Autodesk Inventor part; units mm, degrees
(part 3 of 3)
sketch "Sketch16" plane through (-107.75, 0, 0) normal (0, 0, 1) x (1, 0, 0)
  line L0 (4.2221, 29.7336) -> (86.2779, 29.7336) construction
  line L1 (86.2779, 29.7336) -> (86.2779, 24.45) construction
  line L2 (86.2779, 24.45) -> (4.2221, 24.45) construction
  line L3 (4.2221, 24.45) -> (4.2221, 29.7336) construction
  line L4 (30.85, 22.45) -> (59.65, 22.45) projected
  line L5 (20.4356, 29.4257) -> (17.6446, 29.4257)
  line L6 (17.6446, 29.4257) -> (17.6446, 27.7336)
  line L7 (17.6446, 27.7336) -> (20.3189, 27.7336)
  line L8 (20.3189, 27.7336) -> (20.3189, 27.0237)
  line L9 (20.3189, 27.0237) -> (17.6446, 27.0237)
  line L10 (17.6446, 27.0237) -> (17.6446, 24.1356)
  line L11 (17.6446, 24.1356) -> (16.8472, 24.1356)
  line L12 (16.8472, 24.1356) -> (16.8472, 30.1356)
  line L13 (16.8472, 30.1356) -> (20.4356, 30.1356)
  line L14 (20.4356, 30.1356) -> (20.4356, 29.4257)
  line L15 (23.4793, 27.826) -> (23.4404, 27.826)
  spline S0 degree 2 poles (23.4404, 27.826) (23.3529, 27.8503) (23.1633, 27.86) (23.032, 27.86) knots 0 0 0 1 2 2 2
  spline S1 degree 2 poles (23.032, 27.86) (22.7257, 27.86) (22.1228, 27.5926) (21.8505, 27.3301) knots 0 0 0 1 2 2 2
  line L16 (21.8505, 27.3301) -> (21.8505, 24.1356)
  line L17 (21.8505, 24.1356) -> (21.092, 24.1356)
  line L18 (21.092, 24.1356) -> (21.092, 28.638)
  line L19 (21.092, 28.638) -> (21.8505, 28.638)
  line L20 (21.8505, 28.638) -> (21.8505, 27.967)
  spline S2 degree 2 poles (21.8505, 27.967) (22.2638, 28.3365) (22.8813, 28.638) (23.173, 28.638) knots 0 0 0 1 2 2 2
  spline S3 degree 2 poles (23.173, 28.638) (23.2897, 28.638) (23.4064, 28.6283) (23.4793, 28.6137) knots 0 0 0 1 2 2 2
  line L21 (23.4793, 28.6137) -> (23.4793, 27.826)
  spline S4 degree 2 poles (27.7678, 26.3868) (27.7678, 25.249) (26.6738, 24.0092) (25.7597, 24.0092) knots 0 0 0 1 2 2 2
  spline S5 degree 2 poles (25.7597, 24.0092) (24.8213, 24.0092) (23.7468, 25.2879) (23.7468, 26.3868) knots 0 0 0 1 2 2 2
  spline S6 degree 2 poles (23.7468, 26.3868) (23.7468, 27.5148) (24.8553, 28.7644) (25.7597, 28.7644) knots 0 0 0 1 2 2 2
  spline S7 degree 2 poles (25.7597, 28.7644) (26.6738, 28.7644) (27.7678, 27.5197) (27.7678, 26.3868) knots 0 0 0 1 2 2 2
  spline S8 degree 2 poles (26.985, 26.3868) (26.985, 27.262) (26.3481, 28.1129) (25.7597, 28.1129) knots 0 0 0 1 2 2 2
  spline S9 degree 2 poles (25.7597, 28.1129) (25.1714, 28.1129) (24.5296, 27.262) (24.5296, 26.3868) knots 0 0 0 1 2 2 2
  spline S10 degree 2 poles (24.5296, 26.3868) (24.5296, 25.5359) (25.1714, 24.6607) (25.7597, 24.6607) knots 0 0 0 1 2 2 2
  spline S11 degree 2 poles (25.7597, 24.6607) (26.3432, 24.6607) (26.985, 25.5213) (26.985, 26.3868) knots 0 0 0 1 2 2 2
  line L22 (32.0806, 24.1356) -> (31.3221, 24.1356)
  line L23 (31.3221, 24.1356) -> (31.3221, 26.7028)
  spline S12 degree 2 poles (31.3221, 26.7028) (31.3221, 27.014) (31.2638, 27.5489) (31.1763, 27.7093) knots 0 0 0 1 2 2 2
  spline S13 degree 2 poles (31.1763, 27.7093) (31.0839, 27.8795) (30.7532, 28.0448) (30.4712, 28.0448) knots 0 0 0 1 2 2 2
  spline S14 degree 2 poles (30.4712, 28.0448) (30.1892, 28.0448) (29.5912, 27.7434) (29.3043, 27.5002) knots 0 0 0 1 2 2 2
  line L24 (29.3043, 27.5002) -> (29.3043, 24.1356)
  line L25 (29.3043, 24.1356) -> (28.5458, 24.1356)
  line L26 (28.5458, 24.1356) -> (28.5458, 28.638)
  line L27 (28.5458, 28.638) -> (29.3043, 28.638)
  line L28 (29.3043, 28.638) -> (29.3043, 28.1372)
  spline S15 degree 2 poles (29.3043, 28.1372) (29.6447, 28.4435) (30.3011, 28.7644) (30.6706, 28.7644) knots 0 0 0 1 2 2 2
  spline S16 degree 2 poles (30.6706, 28.7644) (31.3318, 28.7644) (32.0806, 27.8892) (32.0806, 27.0578) knots 0 0 0 1 2 2 2
  line L29 (32.0806, 27.0578) -> (32.0806, 24.1356)
  spline S17 degree 2 poles (34.5069, 24.0481) (33.8894, 24.0481) (33.1941, 24.7531) (33.1941, 25.5165) knots 0 0 0 1 2 2 2
  line L30 (33.1941, 25.5165) -> (33.1941, 28.0108)
  line L31 (33.1941, 28.0108) -> (32.6835, 28.0108)
  line L32 (32.6835, 28.0108) -> (32.6835, 28.638)
  line L33 (32.6835, 28.638) -> (33.1941, 28.638)
  line L34 (33.1941, 28.638) -> (33.1941, 29.9314)
  line L35 (33.1941, 29.9314) -> (33.9526, 29.9314)
  line L36 (33.9526, 29.9314) -> (33.9526, 28.638)
  line L37 (33.9526, 28.638) -> (35.3481, 28.638)
  line L38 (35.3481, 28.638) -> (35.3481, 28.0108)
  line L39 (35.3481, 28.0108) -> (33.9526, 28.0108)
  line L40 (33.9526, 28.0108) -> (33.9526, 25.8665)
  spline S18 degree 2 poles (33.9526, 25.8665) (33.9526, 25.5262) (33.9769, 25.1518) (34.0596, 24.9913) knots 0 0 0 1 2 2 2
  spline S19 degree 2 poles (34.0596, 24.9913) (34.1276, 24.8503) (34.434, 24.7093) (34.6965, 24.7093) knots 0 0 0 1 2 2 2
  spline S20 degree 2 poles (34.6965, 24.7093) (34.8813, 24.7093) (35.2265, 24.8212) (35.3043, 24.8552) knots 0 0 0 1 2 2 2
  line L41 (35.3043, 24.8552) -> (35.3481, 24.8552)
  line L42 (35.3481, 24.8552) -> (35.3481, 24.1745)
  spline S21 degree 2 poles (35.3481, 24.1745) (35.1341, 24.1161) (34.6965, 24.0481) (34.5069, 24.0481) knots 0 0 0 1 2 2 2
  spline S22 degree 2 poles (42.6122, 25.9784) (42.6122, 25.531) (42.2719, 24.8455) (41.9899, 24.6218) knots 0 0 0 1 2 2 2
  spline S23 degree 2 poles (41.9899, 24.6218) (41.6495, 24.3592) (40.8764, 24.1356) (40.2638, 24.1356) knots 0 0 0 1 2 2 2
  line L43 (40.2638, 24.1356) -> (38.5425, 24.1356)
  line L44 (38.5425, 24.1356) -> (38.5425, 30.1356)
  line L45 (38.5425, 30.1356) -> (40.1325, 30.1356)
  spline S24 degree 2 poles (40.1325, 30.1356) (40.7743, 30.1356) (41.4161, 30.0529) (41.7079, 29.8925) knots 0 0 0 1 2 2 2
  spline S25 degree 2 poles (41.7079, 29.8925) (42.0336, 29.7223) (42.3302, 29.1631) (42.3302, 28.7839) knots 0 0 0 1 2 2 2
  spline S26 degree 2 poles (42.3302, 28.7839) (42.3302, 28.3609) (41.8829, 27.6899) (41.4891, 27.5002) knots 0 0 0 1 2 2 2
  line L46 (41.4891, 27.5002) -> (41.4891, 27.4711)
  spline S27 degree 2 poles (41.4891, 27.4711) (42.0239, 27.3252) (42.6122, 26.5521) (42.6122, 25.9784) knots 0 0 0 1 2 2 2
  spline S28 degree 2 poles (41.7808, 25.9443) (41.7808, 26.2847) (41.5863, 26.7223) (41.2946, 26.8779) knots 0 0 0 1 2 2 2
  spline S29 degree 2 poles (41.2946, 26.8779) (41.1049, 26.9751) (40.6576, 27.0335) (40.2443, 27.0335) knots 0 0 0 1 2 2 2
  line L47 (40.2443, 27.0335) -> (39.34, 27.0335)
  line L48 (39.34, 27.0335) -> (39.34, 24.8163)
  line L49 (39.34, 24.8163) -> (39.9866, 24.8163)
  spline S30 degree 2 poles (39.9866, 24.8163) (40.5117, 24.8163) (41.1147, 24.9135) (41.3481, 25.0691) knots 0 0 0 1 2 2 2
  spline S31 degree 2 poles (41.3481, 25.0691) (41.5717, 25.2296) (41.7808, 25.6283) (41.7808, 25.9443) knots 0 0 0 1 2 2 2
  spline S32 degree 2 poles (41.4988, 28.672) (41.4988, 28.886) (41.3529, 29.2069) (41.1925, 29.2993) knots 0 0 0 1 2 2 2
  spline S33 degree 2 poles (41.1925, 29.2993) (40.998, 29.4062) (40.5263, 29.4549) (40.1033, 29.4549) knots 0 0 0 1 2 2 2
  line L50 (40.1033, 29.4549) -> (39.34, 29.4549)
  line L51 (39.34, 29.4549) -> (39.34, 27.6996)
  line L52 (39.34, 27.6996) -> (40.2443, 27.6996)
  spline S34 degree 2 poles (40.2443, 27.6996) (40.6187, 27.6996) (40.9737, 27.7774) (41.1633, 27.8989) knots 0 0 0 1 2 2 2
  spline S35 degree 2 poles (41.1633, 27.8989) (41.3481, 28.0156) (41.4988, 28.39) (41.4988, 28.672) knots 0 0 0 1 2 2 2
  spline S36 degree 2 poles (47.0466, 26.3868) (47.0466, 25.249) (45.9526, 24.0092) (45.0385, 24.0092) knots 0 0 0 1 2 2 2
  spline S37 degree 2 poles (45.0385, 24.0092) (44.1001, 24.0092) (43.0255, 25.2879) (43.0255, 26.3868) knots 0 0 0 1 2 2 2
  spline S38 degree 2 poles (43.0255, 26.3868) (43.0255, 27.5148) (44.1341, 28.7644) (45.0385, 28.7644) knots 0 0 0 1 2 2 2
  spline S39 degree 2 poles (45.0385, 28.7644) (45.9526, 28.7644) (47.0466, 27.5197) (47.0466, 26.3868) knots 0 0 0 1 2 2 2
  spline S40 degree 2 poles (46.2638, 26.3868) (46.2638, 27.262) (45.6268, 28.1129) (45.0385, 28.1129) knots 0 0 0 1 2 2 2
  spline S41 degree 2 poles (45.0385, 28.1129) (44.4502, 28.1129) (43.8083, 27.262) (43.8083, 26.3868) knots 0 0 0 1 2 2 2
  spline S42 degree 2 poles (43.8083, 26.3868) (43.8083, 25.5359) (44.4502, 24.6607) (45.0385, 24.6607) knots 0 0 0 1 2 2 2
  spline S43 degree 2 poles (45.0385, 24.6607) (45.622, 24.6607) (46.2638, 25.5213) (46.2638, 26.3868) knots 0 0 0 1 2 2 2
  line L53 (51.3205, 24.1356) -> (50.3918, 24.1356)
  line L54 (50.3918, 24.1356) -> (49.2978, 25.8276)
  line L55 (49.2978, 25.8276) -> (48.1746, 24.1356)
  line L56 (48.1746, 24.1356) -> (47.314, 24.1356)
  line L57 (47.314, 24.1356) -> (48.8748, 26.3673)
  line L58 (48.8748, 26.3673) -> (47.3286, 28.638)
  line L59 (47.3286, 28.638) -> (48.2573, 28.638)
  line L60 (48.2573, 28.638) -> (49.3464, 26.9605)
  line L61 (49.3464, 26.9605) -> (50.4599, 28.638)
  line L62 (50.4599, 28.638) -> (51.3205, 28.638)
  line L63 (51.3205, 28.638) -> (49.7694, 26.416)
  line L64 (49.7694, 26.416) -> (51.3205, 24.1356)
  line L65 (61.2686, 30.1356) -> (59.7613, 24.1356)
  line L66 (59.7613, 24.1356) -> (58.8667, 24.1356)
  line L67 (58.8667, 24.1356) -> (57.6463, 29.1145)
  line L68 (57.6463, 29.1145) -> (56.4599, 24.1356)
  line L69 (56.4599, 24.1356) -> (55.575, 24.1356)
  line L70 (55.575, 24.1356) -> (54.0434, 30.1356)
  line L71 (54.0434, 30.1356) -> (54.8651, 30.1356)
  line L72 (54.8651, 30.1356) -> (56.0709, 25.1615)
  line L73 (56.0709, 25.1615) -> (57.267, 30.1356)
  line L74 (57.267, 30.1356) -> (58.079, 30.1356)
  line L75 (58.079, 30.1356) -> (59.2848, 25.1032)
  line L76 (59.2848, 25.1032) -> (60.4858, 30.1356)
  line L77 (60.4858, 30.1356) -> (61.2686, 30.1356)
  line L78 (62.6981, 24.1356) -> (61.9396, 24.1356)
  line L79 (61.9396, 24.1356) -> (61.9396, 28.638)
  line L80 (61.9396, 28.638) -> (62.6981, 28.638)
  line L81 (62.6981, 28.638) -> (62.6981, 24.1356)
  line L82 (62.7516, 29.3868) -> (61.891, 29.3868)
  line L83 (61.891, 29.3868) -> (61.891, 30.1745)
  line L84 (61.891, 30.1745) -> (62.7516, 30.1745)
  line L85 (62.7516, 30.1745) -> (62.7516, 29.3868)
  line L86 (66.1989, 27.826) -> (66.16, 27.826)
  spline S44 degree 2 poles (66.16, 27.826) (66.0725, 27.8503) (65.8829, 27.86) (65.7516, 27.86) knots 0 0 0 1 2 2 2
  spline S45 degree 2 poles (65.7516, 27.86) (65.4453, 27.86) (64.8424, 27.5926) (64.5701, 27.3301) knots 0 0 0 1 2 2 2
  line L87 (64.5701, 27.3301) -> (64.5701, 24.1356)
  line L88 (64.5701, 24.1356) -> (63.8116, 24.1356)
  line L89 (63.8116, 24.1356) -> (63.8116, 28.638)
  line L90 (63.8116, 28.638) -> (64.5701, 28.638)
  line L91 (64.5701, 28.638) -> (64.5701, 27.967)
  spline S46 degree 2 poles (64.5701, 27.967) (64.9834, 28.3365) (65.6009, 28.638) (65.8926, 28.638) knots 0 0 0 1 2 2 2
  spline S47 degree 2 poles (65.8926, 28.638) (66.0093, 28.638) (66.126, 28.6283) (66.1989, 28.6137) knots 0 0 0 1 2 2 2
  line L92 (66.1989, 28.6137) -> (66.1989, 27.826)
  spline S48 degree 2 poles (68.7419, 24.0335) (67.6625, 24.0335) (66.4761, 25.2442) (66.4761, 26.3625) knots 0 0 0 1 2 2 2
  spline S49 degree 2 poles (66.4761, 26.3625) (66.4761, 27.4613) (67.6284, 28.7644) (68.5571, 28.7644) knots 0 0 0 1 2 2 2
  spline S50 degree 2 poles (68.5571, 28.7644) (68.9753, 28.7644) (69.622, 28.5213) (69.8602, 28.2636) knots 0 0 0 1 2 2 2
  spline S51 degree 2 poles (69.8602, 28.2636) (70.1033, 28.0059) (70.361, 27.262) (70.361, 26.7223) knots 0 0 0 1 2 2 2
  line L93 (70.361, 26.7223) -> (70.361, 26.309)
  line L94 (70.361, 26.309) -> (67.2443, 26.309)
  spline S52 degree 2 poles (67.2443, 26.309) (67.2443, 25.5262) (68.032, 24.6947) (68.7322, 24.6947) knots 0 0 0 1 2 2 2
  spline S53 degree 2 poles (68.7322, 24.6947) (68.9801, 24.6947) (69.4615, 24.8066) (69.656, 24.8941) knots 0 0 0 1 2 2 2
  spline S54 degree 2 poles (69.656, 24.8941) (69.8602, 24.9913) (70.1422, 25.1615) (70.2346, 25.2393) knots 0 0 0 1 2 2 2
  line L95 (70.2346, 25.2393) -> (70.2784, 25.2393)
  line L96 (70.2784, 25.2393) -> (70.2784, 24.4127)
  spline S55 degree 2 poles (70.2784, 24.4127) (70.1471, 24.3592) (69.7484, 24.2036) (69.5928, 24.1599) knots 0 0 0 1 2 2 2
  spline S56 degree 2 poles (69.5928, 24.1599) (69.374, 24.0967) (69.0142, 24.0335) (68.7419, 24.0335) knots 0 0 0 1 2 2 2
  spline S57 degree 2 poles (69.622, 26.8876) (69.6122, 27.1939) (69.4858, 27.6412) (69.3643, 27.792) knots 0 0 0 1 2 2 2
  spline S58 degree 2 poles (69.3643, 27.792) (69.233, 27.9622) (68.8197, 28.1421) (68.5134, 28.1421) knots 0 0 0 1 2 2 2
  spline S59 degree 2 poles (68.5134, 28.1421) (68.2119, 28.1421) (67.7889, 27.9622) (67.6139, 27.7871) knots 0 0 0 1 2 2 2
  spline S60 degree 2 poles (67.6139, 27.7871) (67.4437, 27.6072) (67.2686, 27.1745) (67.2443, 26.8876) knots 0 0 0 1 2 2 2
  line L97 (67.2443, 26.8876) -> (69.622, 26.8876)
  spline S61 degree 2 poles (72.3448, 24.0286) (71.8926, 24.0286) (71.1098, 24.2717) (70.8521, 24.4079) knots 0 0 0 1 2 2 2
  line L98 (70.8521, 24.4079) -> (70.8521, 25.2588)
  line L99 (70.8521, 25.2588) -> (70.891, 25.2588)
  spline S62 degree 2 poles (70.891, 25.2588) (70.9882, 25.181) (71.2508, 24.9962) (71.4696, 24.8941) knots 0 0 0 1 2 2 2
  spline S63 degree 2 poles (71.4696, 24.8941) (71.6592, 24.8017) (72.126, 24.6656) (72.374, 24.6656) knots 0 0 0 1 2 2 2
  spline S64 degree 2 poles (72.374, 24.6656) (72.5539, 24.6656) (72.9672, 24.7482) (73.0644, 24.8163) knots 0 0 0 1 2 2 2
  spline S65 degree 2 poles (73.0644, 24.8163) (73.2054, 24.9087) (73.3318, 25.1177) (73.3318, 25.3317) knots 0 0 0 1 2 2 2
  spline S66 degree 2 poles (73.3318, 25.3317) (73.3318, 25.5991) (73.0401, 25.8763) (72.6657, 25.9686) knots 0 0 0 1 2 2 2
  spline S67 degree 2 poles (72.6657, 25.9686) (72.5199, 26.0027) (72.0531, 26.0999) (71.8537, 26.1534) knots 0 0 0 1 2 2 2
  spline S68 degree 2 poles (71.8537, 26.1534) (71.3383, 26.3041) (70.8716, 26.9265) (70.8716, 27.369) knots 0 0 0 1 2 2 2
  spline S69 degree 2 poles (70.8716, 27.369) (70.8716, 27.9816) (71.7905, 28.745) (72.549, 28.745) knots 0 0 0 1 2 2 2
  spline S70 degree 2 poles (72.549, 28.745) (72.9234, 28.745) (73.6819, 28.5602) (73.9396, 28.4192) knots 0 0 0 1 2 2 2
  line L100 (73.9396, 28.4192) -> (73.9396, 27.6072)
  line L101 (73.9396, 27.6072) -> (73.9007, 27.6072)
  spline S71 degree 2 poles (73.9007, 27.6072) (73.609, 27.8406) (72.8991, 28.108) (72.5344, 28.108) knots 0 0 0 1 2 2 2
  spline S72 degree 2 poles (72.5344, 28.108) (72.16, 28.108) (71.6447, 27.792) (71.6447, 27.4759) knots 0 0 0 1 2 2 2
  spline S73 degree 2 poles (71.6447, 27.4759) (71.6447, 27.1891) (71.951, 26.9119) (72.2913, 26.8244) knots 0 0 0 1 2 2 2
  spline S74 degree 2 poles (72.2913, 26.8244) (72.4566, 26.7806) (72.8748, 26.6931) (73.1033, 26.6396) knots 0 0 0 1 2 2 2
  spline S75 degree 2 poles (73.1033, 26.6396) (73.5993, 26.5132) (74.1049, 25.9346) (74.1049, 25.4338) knots 0 0 0 1 2 2 2
  spline S76 degree 2 poles (74.1049, 25.4338) (74.1049, 25.1421) (73.8764, 24.6267) (73.6528, 24.437) knots 0 0 0 1 2 2 2
  spline S77 degree 2 poles (73.6528, 24.437) (73.4145, 24.2377) (72.8067, 24.0286) (72.3448, 24.0286) knots 0 0 0 1 2 2 2
  point P0 (107.75, 0)
  point P1 (45.25, 24.45)
  point P2 (45.25, 22.45)
  point P3 (45.25, 22.45)
  dimension "d146" = 0
  dimension "d147" = 2
  constraints: 3 midpoint, 2 other
  measures "d146" horizontal distance of point (45.25, 24.45) point (45.25, 22.45)
  measures "d147" distance of point (45.25, 22.45) point (45.25, 24.45)
sketch "Sketch17" plane through (0, 0, -2.25) normal (1, 0, 0) x (0, 0, -1)
  line L0 (72.0372, 28.5438) -> (116.4628, 28.5438) construction
  line L1 (116.4628, 28.5438) -> (116.4628, 24.45) construction
  line L2 (116.4628, 24.45) -> (72.0372, 24.45) construction
  line L3 (72.0372, 24.45) -> (72.0372, 28.5438) construction
  line L4 (88.9, 22.45) -> (99.6, 22.45) projected
  line L5 (78.0247, 23.5407) -> (77.2273, 23.5407)
  line L6 (77.2273, 23.5407) -> (77.2273, 28.7092)
  line L7 (77.2273, 28.7092) -> (75.6617, 25.1938)
  line L8 (75.6617, 25.1938) -> (75.1754, 25.1938)
  line L9 (75.1754, 25.1938) -> (73.6244, 28.7092)
  line L10 (73.6244, 28.7092) -> (73.6244, 23.5407)
  line L11 (73.6244, 23.5407) -> (72.8805, 23.5407)
  line L12 (72.8805, 23.5407) -> (72.8805, 29.5407)
  line L13 (72.8805, 29.5407) -> (73.9696, 29.5407)
  line L14 (73.9696, 29.5407) -> (75.4672, 26.2003)
  line L15 (75.4672, 26.2003) -> (76.9161, 29.5407)
  line L16 (76.9161, 29.5407) -> (78.0247, 29.5407)
  line L17 (78.0247, 29.5407) -> (78.0247, 23.5407)
  spline S0 degree 2 poles (82.8821, 25.7919) (82.8821, 24.6541) (81.7881, 23.4143) (80.874, 23.4143) knots 0 0 0 1 2 2 2
  spline S1 degree 2 poles (80.874, 23.4143) (79.9356, 23.4143) (78.861, 24.693) (78.861, 25.7919) knots 0 0 0 1 2 2 2
  spline S2 degree 2 poles (78.861, 25.7919) (78.861, 26.9199) (79.9696, 28.1695) (80.874, 28.1695) knots 0 0 0 1 2 2 2
  spline S3 degree 2 poles (80.874, 28.1695) (81.7881, 28.1695) (82.8821, 26.9248) (82.8821, 25.7919) knots 0 0 0 1 2 2 2
  spline S4 degree 2 poles (82.0993, 25.7919) (82.0993, 26.6671) (81.4623, 27.518) (80.874, 27.518) knots 0 0 0 1 2 2 2
  spline S5 degree 2 poles (80.874, 27.518) (80.2857, 27.518) (79.6438, 26.6671) (79.6438, 25.7919) knots 0 0 0 1 2 2 2
  spline S6 degree 2 poles (79.6438, 25.7919) (79.6438, 24.941) (80.2857, 24.0658) (80.874, 24.0658) knots 0 0 0 1 2 2 2
  spline S7 degree 2 poles (80.874, 24.0658) (81.4575, 24.0658) (82.0993, 24.9264) (82.0993, 25.7919) knots 0 0 0 1 2 2 2
  spline S8 degree 2 poles (85.0215, 23.4532) (84.404, 23.4532) (83.7087, 24.1582) (83.7087, 24.9216) knots 0 0 0 1 2 2 2
  line L18 (83.7087, 24.9216) -> (83.7087, 27.4159)
  line L19 (83.7087, 27.4159) -> (83.1981, 27.4159)
  line L20 (83.1981, 27.4159) -> (83.1981, 28.0431)
  line L21 (83.1981, 28.0431) -> (83.7087, 28.0431)
  line L22 (83.7087, 28.0431) -> (83.7087, 29.3365)
  line L23 (83.7087, 29.3365) -> (84.4672, 29.3365)
  line L24 (84.4672, 29.3365) -> (84.4672, 28.0431)
  line L25 (84.4672, 28.0431) -> (85.8626, 28.0431)
  line L26 (85.8626, 28.0431) -> (85.8626, 27.4159)
  line L27 (85.8626, 27.4159) -> (84.4672, 27.4159)
  line L28 (84.4672, 27.4159) -> (84.4672, 25.2716)
  spline S9 degree 2 poles (84.4672, 25.2716) (84.4672, 24.9313) (84.4915, 24.5569) (84.5741, 24.3964) knots 0 0 0 1 2 2 2
  spline S10 degree 2 poles (84.5741, 24.3964) (84.6422, 24.2554) (84.9485, 24.1144) (85.2111, 24.1144) knots 0 0 0 1 2 2 2
  spline S11 degree 2 poles (85.2111, 24.1144) (85.3959, 24.1144) (85.7411, 24.2263) (85.8189, 24.2603) knots 0 0 0 1 2 2 2
  line L29 (85.8189, 24.2603) -> (85.8626, 24.2603)
  line L30 (85.8626, 24.2603) -> (85.8626, 23.5796)
  spline S12 degree 2 poles (85.8626, 23.5796) (85.6487, 23.5212) (85.2111, 23.4532) (85.0215, 23.4532) knots 0 0 0 1 2 2 2
  spline S13 degree 2 poles (90.122, 25.7919) (90.122, 24.6541) (89.028, 23.4143) (88.1139, 23.4143) knots 0 0 0 1 2 2 2
  spline S14 degree 2 poles (88.1139, 23.4143) (87.1754, 23.4143) (86.1009, 24.693) (86.1009, 25.7919) knots 0 0 0 1 2 2 2
  spline S15 degree 2 poles (86.1009, 25.7919) (86.1009, 26.9199) (87.2095, 28.1695) (88.1139, 28.1695) knots 0 0 0 1 2 2 2
  spline S16 degree 2 poles (88.1139, 28.1695) (89.028, 28.1695) (90.122, 26.9248) (90.122, 25.7919) knots 0 0 0 1 2 2 2
  spline S17 degree 2 poles (89.3391, 25.7919) (89.3391, 26.6671) (88.7022, 27.518) (88.1139, 27.518) knots 0 0 0 1 2 2 2
  spline S18 degree 2 poles (88.1139, 27.518) (87.5255, 27.518) (86.8837, 26.6671) (86.8837, 25.7919) knots 0 0 0 1 2 2 2
  spline S19 degree 2 poles (86.8837, 25.7919) (86.8837, 24.941) (87.5255, 24.0658) (88.1139, 24.0658) knots 0 0 0 1 2 2 2
  spline S20 degree 2 poles (88.1139, 24.0658) (88.6973, 24.0658) (89.3391, 24.9264) (89.3391, 25.7919) knots 0 0 0 1 2 2 2
  line L31 (93.2873, 27.2311) -> (93.2484, 27.2311)
  spline S21 degree 2 poles (93.2484, 27.2311) (93.1609, 27.2554) (92.9712, 27.2652) (92.84, 27.2652) knots 0 0 0 1 2 2 2
  spline S22 degree 2 poles (92.84, 27.2652) (92.5336, 27.2652) (91.9307, 26.9977) (91.6584, 26.7352) knots 0 0 0 1 2 2 2
  line L32 (91.6584, 26.7352) -> (91.6584, 23.5407)
  line L33 (91.6584, 23.5407) -> (90.8999, 23.5407)
  line L34 (90.8999, 23.5407) -> (90.8999, 28.0431)
  line L35 (90.8999, 28.0431) -> (91.6584, 28.0431)
  line L36 (91.6584, 28.0431) -> (91.6584, 27.3721)
  spline S23 degree 2 poles (91.6584, 27.3721) (92.0717, 27.7417) (92.6892, 28.0431) (92.981, 28.0431) knots 0 0 0 1 2 2 2
  spline S24 degree 2 poles (92.981, 28.0431) (93.0977, 28.0431) (93.2143, 28.0334) (93.2873, 28.0188) knots 0 0 0 1 2 2 2
  line L37 (93.2873, 28.0188) -> (93.2873, 27.2311)
  line L38 (103.2354, 29.5407) -> (101.7281, 23.5407)
  line L39 (101.7281, 23.5407) -> (100.8335, 23.5407)
  line L40 (100.8335, 23.5407) -> (99.613, 28.5196)
  line L41 (99.613, 28.5196) -> (98.4267, 23.5407)
  line L42 (98.4267, 23.5407) -> (97.5417, 23.5407)
  line L43 (97.5417, 23.5407) -> (96.0101, 29.5407)
  line L44 (96.0101, 29.5407) -> (96.8318, 29.5407)
  line L45 (96.8318, 29.5407) -> (98.0377, 24.5666)
  line L46 (98.0377, 24.5666) -> (99.2338, 29.5407)
  line L47 (99.2338, 29.5407) -> (100.0458, 29.5407)
  line L48 (100.0458, 29.5407) -> (101.2516, 24.5083)
  line L49 (101.2516, 24.5083) -> (102.4526, 29.5407)
  line L50 (102.4526, 29.5407) -> (103.2354, 29.5407)
  line L51 (104.6649, 23.5407) -> (103.9064, 23.5407)
  line L52 (103.9064, 23.5407) -> (103.9064, 28.0431)
  line L53 (103.9064, 28.0431) -> (104.6649, 28.0431)
  line L54 (104.6649, 28.0431) -> (104.6649, 23.5407)
  line L55 (104.7184, 28.7919) -> (103.8578, 28.7919)
  line L56 (103.8578, 28.7919) -> (103.8578, 29.5796)
  line L57 (103.8578, 29.5796) -> (104.7184, 29.5796)
  line L58 (104.7184, 29.5796) -> (104.7184, 28.7919)
  line L59 (108.1657, 27.2311) -> (108.1268, 27.2311)
  spline S25 degree 2 poles (108.1268, 27.2311) (108.0393, 27.2554) (107.8497, 27.2652) (107.7184, 27.2652) knots 0 0 0 1 2 2 2
  spline S26 degree 2 poles (107.7184, 27.2652) (107.4121, 27.2652) (106.8092, 26.9977) (106.5369, 26.7352) knots 0 0 0 1 2 2 2
  line L60 (106.5369, 26.7352) -> (106.5369, 23.5407)
  line L61 (106.5369, 23.5407) -> (105.7784, 23.5407)
  line L62 (105.7784, 23.5407) -> (105.7784, 28.0431)
  line L63 (105.7784, 28.0431) -> (106.5369, 28.0431)
  line L64 (106.5369, 28.0431) -> (106.5369, 27.3721)
  spline S27 degree 2 poles (106.5369, 27.3721) (106.9502, 27.7417) (107.5677, 28.0431) (107.8594, 28.0431) knots 0 0 0 1 2 2 2
  spline S28 degree 2 poles (107.8594, 28.0431) (107.9761, 28.0431) (108.0928, 28.0334) (108.1657, 28.0188) knots 0 0 0 1 2 2 2
  line L65 (108.1657, 28.0188) -> (108.1657, 27.2311)
  spline S29 degree 2 poles (110.7087, 23.4386) (109.6293, 23.4386) (108.4429, 24.6493) (108.4429, 25.7676) knots 0 0 0 1 2 2 2
  spline S30 degree 2 poles (108.4429, 25.7676) (108.4429, 26.8665) (109.5952, 28.1695) (110.5239, 28.1695) knots 0 0 0 1 2 2 2
  spline S31 degree 2 poles (110.5239, 28.1695) (110.9421, 28.1695) (111.5887, 27.9264) (111.827, 27.6687) knots 0 0 0 1 2 2 2
  spline S32 degree 2 poles (111.827, 27.6687) (112.0701, 27.411) (112.3278, 26.6671) (112.3278, 26.1274) knots 0 0 0 1 2 2 2
  line L66 (112.3278, 26.1274) -> (112.3278, 25.7141)
  line L67 (112.3278, 25.7141) -> (109.2111, 25.7141)
  spline S33 degree 2 poles (109.2111, 25.7141) (109.2111, 24.9313) (109.9988, 24.0998) (110.6989, 24.0998) knots 0 0 0 1 2 2 2
  spline S34 degree 2 poles (110.6989, 24.0998) (110.9469, 24.0998) (111.4283, 24.2117) (111.6228, 24.2992) knots 0 0 0 1 2 2 2
  spline S35 degree 2 poles (111.6228, 24.2992) (111.827, 24.3964) (112.109, 24.5666) (112.2014, 24.6444) knots 0 0 0 1 2 2 2
  line L68 (112.2014, 24.6444) -> (112.2451, 24.6444)
  line L69 (112.2451, 24.6444) -> (112.2451, 23.8178)
  spline S36 degree 2 poles (112.2451, 23.8178) (112.1139, 23.7643) (111.7152, 23.6088) (111.5596, 23.565) knots 0 0 0 1 2 2 2
  spline S37 degree 2 poles (111.5596, 23.565) (111.3408, 23.5018) (110.981, 23.4386) (110.7087, 23.4386) knots 0 0 0 1 2 2 2
  spline S38 degree 2 poles (111.5887, 26.2927) (111.579, 26.599) (111.4526, 27.0464) (111.331, 27.1971) knots 0 0 0 1 2 2 2
  spline S39 degree 2 poles (111.331, 27.1971) (111.1998, 27.3673) (110.7865, 27.5472) (110.4801, 27.5472) knots 0 0 0 1 2 2 2
  spline S40 degree 2 poles (110.4801, 27.5472) (110.1787, 27.5472) (109.7557, 27.3673) (109.5806, 27.1922) knots 0 0 0 1 2 2 2
  spline S41 degree 2 poles (109.5806, 27.1922) (109.4105, 27.0123) (109.2354, 26.5796) (109.2111, 26.2927) knots 0 0 0 1 2 2 2
  line L70 (109.2111, 26.2927) -> (111.5887, 26.2927)
  spline S42 degree 2 poles (114.3116, 23.4337) (113.8594, 23.4337) (113.0766, 23.6768) (112.8189, 23.813) knots 0 0 0 1 2 2 2
  line L71 (112.8189, 23.813) -> (112.8189, 24.6639)
  line L72 (112.8189, 24.6639) -> (112.8578, 24.6639)
  spline S43 degree 2 poles (112.8578, 24.6639) (112.955, 24.5861) (113.2176, 24.4013) (113.4364, 24.2992) knots 0 0 0 1 2 2 2
  spline S44 degree 2 poles (113.4364, 24.2992) (113.626, 24.2068) (114.0928, 24.0707) (114.3408, 24.0707) knots 0 0 0 1 2 2 2
  spline S45 degree 2 poles (114.3408, 24.0707) (114.5207, 24.0707) (114.934, 24.1533) (115.0312, 24.2214) knots 0 0 0 1 2 2 2
  spline S46 degree 2 poles (115.0312, 24.2214) (115.1722, 24.3138) (115.2986, 24.5229) (115.2986, 24.7368) knots 0 0 0 1 2 2 2
  spline S47 degree 2 poles (115.2986, 24.7368) (115.2986, 25.0042) (115.0069, 25.2814) (114.6325, 25.3737) knots 0 0 0 1 2 2 2
  spline S48 degree 2 poles (114.6325, 25.3737) (114.4866, 25.4078) (114.0199, 25.505) (113.8205, 25.5585) knots 0 0 0 1 2 2 2
  spline S49 degree 2 poles (113.8205, 25.5585) (113.3051, 25.7092) (112.8383, 26.3316) (112.8383, 26.7741) knots 0 0 0 1 2 2 2
  spline S50 degree 2 poles (112.8383, 26.7741) (112.8383, 27.3867) (113.7573, 28.1501) (114.5158, 28.1501) knots 0 0 0 1 2 2 2
  spline S51 degree 2 poles (114.5158, 28.1501) (114.8902, 28.1501) (115.6487, 27.9653) (115.9064, 27.8243) knots 0 0 0 1 2 2 2
  line L73 (115.9064, 27.8243) -> (115.9064, 27.0123)
  line L74 (115.9064, 27.0123) -> (115.8675, 27.0123)
  spline S52 degree 2 poles (115.8675, 27.0123) (115.5758, 27.2457) (114.8659, 27.5131) (114.5012, 27.5131) knots 0 0 0 1 2 2 2
  spline S53 degree 2 poles (114.5012, 27.5131) (114.1268, 27.5131) (113.6114, 27.1971) (113.6114, 26.881) knots 0 0 0 1 2 2 2
  spline S54 degree 2 poles (113.6114, 26.881) (113.6114, 26.5942) (113.9177, 26.317) (114.2581, 26.2295) knots 0 0 0 1 2 2 2
  spline S55 degree 2 poles (114.2581, 26.2295) (114.4234, 26.1857) (114.8416, 26.0982) (115.0701, 26.0447) knots 0 0 0 1 2 2 2
  spline S56 degree 2 poles (115.0701, 26.0447) (115.566, 25.9183) (116.0717, 25.3397) (116.0717, 24.8389) knots 0 0 0 1 2 2 2
  spline S57 degree 2 poles (116.0717, 24.8389) (116.0717, 24.5472) (115.8432, 24.0318) (115.6195, 23.8421) knots 0 0 0 1 2 2 2
  spline S58 degree 2 poles (115.6195, 23.8421) (115.3813, 23.6428) (114.7735, 23.4337) (114.3116, 23.4337) knots 0 0 0 1 2 2 2
  point P0 (-2.25, 0)
  point P1 (94.25, 24.45)
  point P2 (94.25, 22.45)
  point P3 (94.25, 22.45)
  dimension "d148" = 2
  dimension "d149" = 0
  constraints: 3 midpoint, 2 other
  measures "d148" distance of point (94.25, 24.45) point (94.25, 22.45)
  measures "d149" horizontal distance of point (94.25, 24.45) point (94.25, 22.45)
extrude "Extrusion15" cut sketch "Sketch14" against normal blind 1.5 contours S0 S1 L5 L6 L7 S2 S3 S4 L8 S5 | S14 S15 S16 S17 S18 S19 L15 S20 S21 S22 L16 L17 S23 S24 S25 L18 L19 L20 | L22 S30 S31 L23 L24 L25 L26 L27 S32 S33 L28 | L29 S34 S35 L30 L31 L32 L33 L34 S36 S37 L35 | S38 S39 S40 S41 L36 L37 S42 S43 S44 L38 L39 S45 S46 | L41 L42 L43 L44 | S51 S52 L45 L46 L47 L48 L49 S53 S54 | S59 S60 S61 S62 | L53 L54 L55 L56 L57 L58 L59 L60 L61 L62 L63 L64 L65 | S67 S68 S69 S70 L66 L67 S71 S72 S73 L68 L69 S74 S75 | L71 S80 S81 L72 L73 L74 L75 L76 S82 S83 L77 | S84 S85 L78 L79 L80 L81 L82 S86 S87 | S92 S93 S94 S95 | L86 S100 S101 L87 L88 L89 L90 L91 S102 S103 L92 | S104 L93 L94 L95 L96 L97 L98 L99 L100 L101 L102 L103 S105 S106 S107 L104 L105 S108
extrude "Extrusion16" cut sketch "Sketch15" against normal blind 1.5
extrude "Extrusion17" cut sketch "Sketch17" against normal blind 1.5
extrude "Extrusion18" cut sketch "Sketch16" against normal blind 1.5
body "Solid1"
